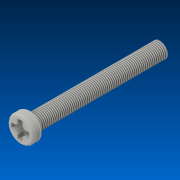
# Autodesk Inventor part: Parafuso lateral do captador
Saved by Autodesk Inventor 2016 (Build 200138000, 138)
## iProperties
Created: 2018-12-10
Part Number: Parafuso lateral do captador
Material: Generic
Document SubType Name: Modeling
Designer: lesly
Density: 1 g/cm^3
Appearance: Default
Author: lesly
Autodesk Inventor part; units mm, degrees
ref_plane "YZ Plane" through (0, 0, 0) normal (1, 0, 0) x (0, 1, 0)
ref_plane "XZ Plane" through (0, 0, 0) normal (0, 1, 0) x (-1, 0, 0)
ref_plane "XY Plane" through (0, 0, 0) normal (0, 0, 1) x (1, 0, 0)
sketch "Sketch1" plane through (0, 0, 0) normal (1, 0, 0) x (0, 1, 0)
  circle A0 centre (0, 0) radius 1.5
  dimension "d0" = 3
  constraints: 1 centre point, 1 coincident
  measures "d0" diameter of A0
extrude "Extrusion1" add sketch "Sketch1" against normal blind 25
sketch "Sketch2" plane through (0, 0, 0) normal (1, 0, 0) x (0, 0, -1)
  circle A0 centre (0, 0) radius 2.5
  dimension "d3" = 5
  constraints: 1 centre point, 1 coincident
  measures "d3" diameter of A0
extrude "Extrusion2" add sketch "Sketch2" along normal blind 2
fillet "Fillet1" radius 0.5 2 edges at (0, 0, 2.5) (2, 0, 2.5)
sketch "Sketch3" plane through (2, 0, 0) normal (1, 0, 0) x (0, 0, -1)
  line L0 (1.75, -0.5) -> (1.75, 0.5)
  line L1 (-1.75, 0.5) -> (-1.75, -0.5)
  line L2 (0.5, 1.75) -> (-0.5, 1.75)
  line L3 (-0.5, -1.75) -> (0.5, -1.75)
  line L4 (-0.5, 1.75) -> (-0.5, 0.866)
  line L5 (-0.5, -0.866) -> (-0.5, -1.75)
  line L6 (-1.75, -0.5) -> (-0.866, -0.5)
  line L7 (0.866, -0.5) -> (1.75, -0.5)
  line L8 (1.75, 0.5) -> (0.866, 0.5)
  line L9 (-0.866, 0.5) -> (-1.75, 0.5)
  line L10 (0.5, -1.75) -> (0.5, -0.866)
  line L11 (0.5, 0.866) -> (0.5, 1.75)
  arc A0 (-0.5, 0.866) -> (-0.866, 0.5) centre (0, 0) ccw
  arc A1 (-0.866, -0.5) -> (-0.5, -0.866) centre (0, 0) ccw
  arc A2 (0.5, -0.866) -> (0.866, -0.5) centre (0, 0) ccw
  arc A3 (0.866, 0.5) -> (0.5, 0.866) centre (0, 0) ccw
  dimension "d7" = 3.5
  dimension "d8" = 1
  dimension "d9" = 3.5
  dimension "d10" = 1
  constraints: 24 end point, 10 parallel, 8 point on circle, 4 centre point, 4 perpendicular, 2 horizontal
  measures "d7" distance of L1.start L0.end
  measures "d8" distance of L0.end L0.start
  measures "d9" distance of L3.start L2.end
  measures "d10" distance of L2.end L2.start
extrude "Extrusion3" cut sketch "Sketch3" against normal blind 1.2
thread "Thread1" size "M3x0.35" class "6g" standard "ANSI Metric M Profile" full length
body "Solid1"
